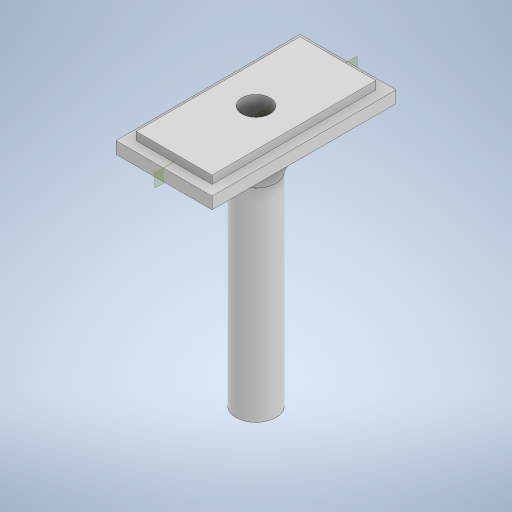
# Autodesk Inventor part: Tampa Eletroimã
Saved by Autodesk Inventor 2023 (Build 270158000, 158)
## iProperties
Created: 2023-03-07
Part Number: Tampa Eletroimã
Material: Genérico
Document SubType Name: Modeling
Designer: Inteli
Density: 1 g/cm^3
Appearance: Padrão
Author: Inteli
Autodesk Inventor part; units mm, degrees
ref_plane "YZ Plane" through (0, 0, 0) normal (1, 0, 0) x (0, 1, 0)
ref_plane "XZ Plane" through (0, 0, 0) normal (0, 1, 0) x (-1, 0, 0)
ref_plane "XY Plane" through (0, 0, 0) normal (0, 0, 1) x (1, 0, 0)
sketch "Esboço1" plane through (0, 0, 0) normal (0, 1, 0) x (-1, 0, 0)
  line L0 (12, 23) -> (-12, 23)
  line L1 (-12, 23) -> (-12, -23)
  line L2 (-12, -23) -> (12, -23)
  line L3 (12, -23) -> (12, 23)
  line L4 (12, 23) -> (-12, -23) construction
  line L5 (-12, 23) -> (12, -23) construction
  point P0 (0, 0)
  dimension "d0" = 24
  dimension "d1" = 46
  constraints: 12 end point, 2 midpoint, 2 parallel, 1 horizontal, 1 perpendicular
  measures "d0" distance of L2.end L1.end
  measures "d1" distance of L1.end L0.end
extrude "Base" add sketch "Esboço1" along normal blind 3
sketch "Esboço2" plane through (0, 3, 0) normal (0, 1, 0) x (1, 0, 0)
  line L0 (-9.5, -20.5) -> (9.5, -20.5)
  line L1 (9.5, -20.5) -> (9.5, 20.5)
  line L2 (9.5, 20.5) -> (-9.5, 20.5)
  line L3 (-9.5, 20.5) -> (-9.5, -20.5)
  line L4 (-9.5, -20.5) -> (9.5, 20.5) construction
  line L5 (9.5, -20.5) -> (-9.5, 20.5) construction
  line L6 (-12, 23) -> (-12, -23) projected
  point P0 (0, 0)
  dimension "d4" = 19
  dimension "d5" = 41
  constraints: 12 end point, 2 midpoint, 2 parallel, 1 horizontal, 1 perpendicular
  measures "d4" distance of L2.end L1.end
  measures "d5" distance of L1.end L0.end
extrude "Encaixe" add sketch "Esboço2" along normal blind 2
sketch "Esboço3" plane through (0, 0, 0) normal (0, -1, 0) x (1, 0, 0)
  circle A0 centre (0, 0) radius 5
  circle A1 centre (0, 0) radius 3.5
  dimension "d9" = 10
  dimension "d10" = 7
  constraints: 2 centre point, 2 coincident
  measures "d9" diameter of A0
  measures "d10" diameter of A1
extrude "Furo" cut sketch "Esboço3" against normal up to surface (5 mm away) contours A1
extrude "Haste" add sketch "Esboço3" along normal blind 60
ref_plane "Plano de trabalho1" through (0, 0, -23) normal (-1, 0, 0) x (0, 0, 1)
sketch "Esboço5" plane through (0, 0, -23) normal (-1, 0, 0) x (0, 0, 1)
  line L0 (18.5938, -14.3413) -> (18.5938, 1.7927)
  line L1 (46, 0) -> (0, 0) projected
  line L2 (26.5, -60) -> (26.5, 5) projected
  arc A0 (18.5938, -14.3413) -> (11, 0) centre (2.6099, -13.6237) ccw
  line L3 (23, -21.6532) -> (23, 7.4929)
  line L4 (0, 0) -> (46, 0) projected
  point P0 (23, 0)
  point P1 (26.9955, 0)
  point P2 (23, 0)
  point P3 (23, 0)
  point P4 (18.5938, -12.9061)
  point P5 (18.5938, 0)
  dimension "d25" = 16
  dimension "d27" = 12
  constraints: 4 end point, 2 coincident, 2 point on circle, 1 centre point, 1 vertical, 4 other
  measures "d25" radius of A0
  measures "d27" distance of point (11, 0) point (23, 0)
revolve "Revolução1" add sketch "Esboço5" angle 360 about axis through (0, -21.6532, 0) along (0, 1, 0) contours A0 L1 L0
